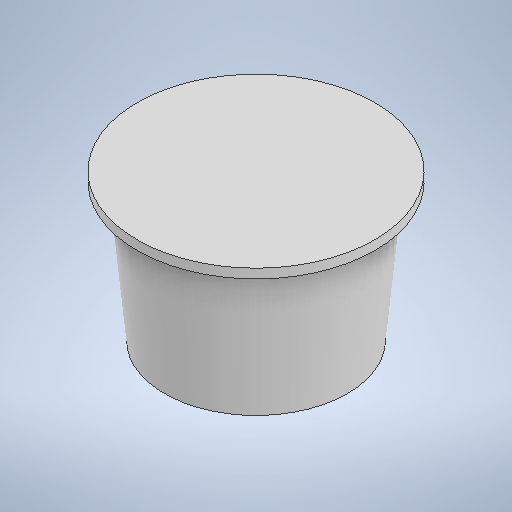
# Autodesk Inventor part: rubberFeet
Saved by Autodesk Inventor 2025 (Build 290162000, 162)
## iProperties
Created: 2026-05-29
Part Number: rubberFeet
Material: Generic
Document SubType Name: Modeling
Designer: tapen
Density: 1 g/cm^3
Appearance: Default
Author: tapen
Autodesk Inventor part; units mm, degrees
ref_plane "YZ Plane" through (0, 0, 0) normal (1, 0, 0) x (0, 1, 0)
ref_plane "XZ Plane" through (0, 0, 0) normal (0, 1, 0) x (-1, 0, 0)
ref_plane "XY Plane" through (0, 0, 0) normal (0, 0, 1) x (1, 0, 0)
sketch "Sketch1" plane through (0, 0, 0) normal (0, 0, 1) x (1, 0, 0)
  line L0 (0, 10.2) -> (8.25, 10.2)
  line L1 (0, 0) -> (6.35, 0)
  line L2 (6.35, 0) -> (7.2484, 9.5537)
  line L3 (7.2484, 9.5537) -> (8.25, 9.5537)
  line L4 (8.25, 9.5537) -> (8.25, 10.2)
  line L5 (0, 0) -> (0, 10.2)
  dimension "d0" = 8.25
  dimension "d1" = 6.35
  dimension "d2" = 10.2
  constraints: 12 end point, 3 horizontal, 2 perpendicular
  measures "d0" distance of L0.start L0.end
  measures "d1" distance of L1.start L1.end
  measures "d2" distance between parallel lines of L1 L0
revolve "Revolution1" add sketch "Sketch1" angle 360 about axis through (0, 0, 0) along (0, 1, 0)
body "Solid1"
